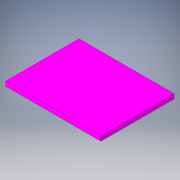
# Autodesk Inventor part: Hombro_tapas
Saved by Autodesk Inventor 2019 (Build 230136000, 136)
## iProperties
Created: 2020-02-08
Part Number: Hombro_tapas
Material: Generic
Document SubType Name: Modeling
Designer: Omar
Density: 1 g/cm^3
Appearance: Default
Author: Omar
Autodesk Inventor part; units mm, degrees
ref_plane "YZ Plane" through (0, 0, 0) normal (1, 0, 0) x (0, 1, 0)
ref_plane "XZ Plane" through (0, 0, 0) normal (0, 1, 0) x (-1, 0, 0)
ref_plane "XY Plane" through (0, 0, 0) normal (0, 0, 1) x (1, 0, 0)
sketch "Sketch1" plane through (0, 0, 0) normal (0, 1, 0) x (-1, 0, 0)
  line L0 (-32.5, 25) -> (32.5, 25)
  line L1 (32.5, 25) -> (32.5, -25)
  line L2 (32.5, -25) -> (-32.5, -25)
  line L3 (-32.5, -25) -> (-32.5, 25)
  line L4 (-32.5, 25) -> (32.5, -25) construction
  line L5 (32.5, 25) -> (-32.5, -25) construction
  point P0 (0, 0)
  dimension "d0" = 65
  dimension "d1" = 50
  constraints: 12 end point, 2 midpoint, 2 parallel, 1 horizontal, 1 perpendicular
  measures "d0" distance of L1.end L2.end
  measures "d1" distance of L0.end L1.end
extrude "Extrusion1" add sketch "Sketch1" along normal blind 3.18
body "Solid1"
